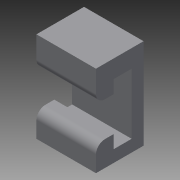
# Autodesk Inventor part: guia
Saved by Autodesk Inventor 2015 SP1 (Build 190203100, 203)
## iProperties
Created: 2015-12-20
Part Number: guia
Material: Generic
Document SubType Name: Modeling
Designer: pc
Density: 1 g/cm^3
Appearance: Default
Author: pc
Autodesk Inventor part; units mm, degrees
ref_plane "YZ Plane" through (0, 0, 0) normal (1, 0, 0) x (0, 1, 0)
ref_plane "XZ Plane" through (0, 0, 0) normal (0, 1, 0) x (-1, 0, 0)
ref_plane "XY Plane" through (0, 0, 0) normal (0, 0, 1) x (1, 0, 0)
sketch "Sketch4" plane through (0, 0, 0) normal (1, 0, 0) x (0, 1, 0)
  line L0 (6, 8) -> (3, 8)
  line L1 (3, 8) -> (3, 5.8)
  line L2 (3, 5.8) -> (0, 5.8)
  line L3 (0, 0) -> (3, 0)
  line L4 (3, 0) -> (3, -2.2)
  line L5 (3, -2.2) -> (6, -2.2)
  line L6 (6, -2.2) -> (6, 8)
  line L7 (8, 11) -> (0, 11)
  line L8 (0, 11) -> (0, 7.8)
  line L9 (0, 7.8) -> (0, 7.8)
  line L10 (0, -4.2) -> (8, -4.2)
  line L11 (8, -4.2) -> (8, 11)
  line L12 (0, 7.8) -> (0, 5.8)
  line L13 (0.2401, 0) -> (0, 0)
  line L14 (0, 0) -> (0, -4.2)
  point P0 (4.5, 8)
  dimension "d23" = 2.2
  dimension "d24" = 3
  dimension "d28" = 2
  dimension "d29" = 5.8
  dimension "d31" = 3
  dimension "d32" = 2
  constraints: 30 end point, 3 collinear, 3 horizontal, 3 point on line, 3 vertical, 1 coincident, 1 horizontal alignment, 1 midpoint, 1 other
  measures "d23" distance of L0.end L1.end
  measures "d24" distance of L0.start L0.end
  measures "d28" distance between parallel lines of L11 L6
  measures "d29" distance of L3.start L2.end
  measures "d31" distance of L1.end L2.end
  measures "d32" distance between parallel lines of L2 L9
extrude "Extrusion3" add sketch "Sketch4" along normal blind 10
fillet "Fillet6" radius 1.5 2 edges at (5, 0, 5.8) (5, 0, 0)
body "Solid2"
